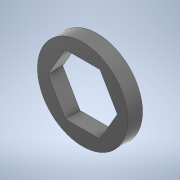
# Autodesk Inventor part: Hex Spacer STOCK
Saved by Autodesk Inventor 2020 (Build 240168000, 168)
## iProperties
Created: 2020-01-16
Part Number: Hex Spacer STOCK
Material: Acetal Resin, Black
Document SubType Name: Modeling
Designer: aidan
Density: 1.425 g/cm^3
Appearance: Smooth - Black
Author: aidan
Autodesk Inventor part; units mm, degrees
ref_plane "YZ Plane" through (0, 0, 0) normal (1, 0, 0) x (0, 1, 0)
ref_plane "XZ Plane" through (0, 0, 0) normal (0, 1, 0) x (-1, 0, 0)
ref_plane "XY Plane" through (0, 0, 0) normal (0, 0, 1) x (1, 0, 0)
sketch "Sketch1" plane through (0, 0, 0) normal (0, 0, 1) x (1, 0, 0)
  line L0 (-7.479, 0) -> (-3.7395, 6.477)
  line L1 (-3.7395, 6.477) -> (3.7395, 6.477)
  line L2 (3.7395, 6.477) -> (7.479, 0)
  line L3 (7.479, 0) -> (3.7395, -6.477)
  line L4 (3.7395, -6.477) -> (-3.7395, -6.477)
  line L5 (-3.7395, -6.477) -> (-7.479, 0)
  circle A0 centre (0, 0) radius 9.7536
  dimension "d0" = 12.954
  dimension "d1" = 19.5072
  constraints: 12 end point, 2 coincident, 1 centre point, 1 horizontal, 13 other
  measures "d0" distance between parallel lines of L1 L4
  measures "d1" diameter of A0
extrude "Extrusion1" add sketch "Sketch1" along normal blind 3.175
equation "\"d3\" = d2"
equation "\"d2\" = 3.175"
body "Solid1"
